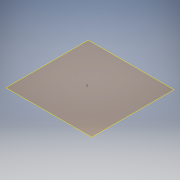
# Autodesk Inventor part: tbe
Saved by Autodesk Inventor 2019 (Build 230136000, 136)
## iProperties
Created: 2019-12-05
Part Number: tbe
Material: Generic
Document SubType Name: Modeling
Designer: Administrator
Density: 1 g/cm^3
Appearance: Default
Author: Administrator
Autodesk Inventor part; units mm, degrees
ref_plane "YZ Plane" through (0, 0, 0) normal (1, 0, 0) x (0, 1, 0)
ref_plane "XZ Plane" through (0, 0, 0) normal (0, 1, 0) x (-1, 0, 0)
ref_plane "XY Plane" through (0, 0, 0) normal (0, 0, 1) x (1, 0, 0)
ref_plane "Work Plane1" through (1030.6797, 97.873, -691.0283) normal (0, 1, 0) x (-1, 0, 0)
sketch "Sketch1" plane through (1030.6797, 97.873, -691.0283) normal (0, 1, 0) x (-1, 0, 0)
  circle A0 centre (729.8421, -338.7609) radius 25.4
  point P0 (1030.6797, 691.0283)
  dimension "d0" = 50.8
  constraints: 1 centre point
  measures "d0" diameter of A0
extrude "Extrusion1" add sketch "Sketch1" against normal blind 381
body "Solid1"
